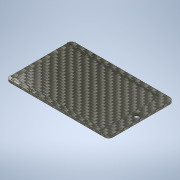
# Autodesk Inventor part: magnet card bottom
Saved by Autodesk Inventor 2020 (Build 240168000, 168)
## iProperties
Created: 2019-06-07
Part Number: magnet card bottom
Material: Generic
Document SubType Name: Modeling
Designer: kangh
Density: 1 g/cm^3
Appearance: Carbon Fiber 1
Author: kangh
Autodesk Inventor part; units mm, degrees
ref_plane "YZ Plane" through (0, 0, 0) normal (1, 0, 0) x (0, 1, 0)
ref_plane "XZ Plane" through (0, 0, 0) normal (0, 1, 0) x (-1, 0, 0)
ref_plane "XY Plane" through (0, 0, 0) normal (0, 0, 1) x (1, 0, 0)
sketch "Sketch1" plane through (0, 0, 0) normal (0, 1, 0) x (-1, 0, 0)
  line L0 (0, 0) -> (85.6, 0)
  line L1 (85.6, 0) -> (85.6, 53.98)
  line L2 (85.6, 53.98) -> (0, 53.98)
  line L3 (0, 53.98) -> (0, 0)
  line L4 (0, 53.98) -> (0, 50.8)
  line L5 (0, 50.8) -> (3.18, 50.8)
  circle A0 centre (3.18, 50.8) radius 3.18
  line L6 (85.6, 53.98) -> (85.6, 57.98)
  line L7 (85.6, 57.98) -> (0, 57.98)
  line L8 (0, 57.98) -> (-9, 57.98)
  line L9 (-9, 57.98) -> (-9, 0)
  line L10 (-9, 0) -> (0, 0)
  line L11 (0, 26.99) -> (-4.5, 26.99)
  circle A1 centre (-4.5, 26.99) radius 2.5
  line L12 (85.6, 55.98) -> (65.6, 55.98)
  circle A2 centre (65.6, 55.98) radius 1
  line L13 (0, 26.99) -> (85.6, 26.99)
  line L14 (85.6, -4) -> (0, -4)
  line L15 (0, -4) -> (-9, -4)
  circle A3 centre (65.6, -2) radius 1
  line L16 (85.6, -4) -> (85.6, 0)
  line L17 (-9, -4) -> (-9, 0)
  line L18 (85.6, 57.98) -> (88.6, 57.98)
  line L19 (88.6, 57.98) -> (88.6, -4)
  line L20 (88.6, -4) -> (85.6, -4)
  line L21 (85.6, -4) -> (85.6, 57.98)
  line L22 (85.6, 53.98) -> (88.6, 53.98)
  line L23 (85.6, 0) -> (88.6, 0)
  circle A4 centre (3.18, 3.18) radius 3.18
  point P0 (3.18, 0)
  point P1 (0, 3.18)
  point P2 (3.18, 53.98)
  dimension "d0" = 85.6
  dimension "d1" = 53.98
  dimension "d2" = 3.18
  dimension "d3" = 3.18
  dimension "d4" = 4
  dimension "d5" = 9
  dimension "d6" = 5
  dimension "d7" = 20
  dimension "d8" = 2
  dimension "d9" = 3
  constraints: 48 end point, 9 perpendicular, 6 point on line, 5 parallel, 5 symmetric about line, 4 centre point, 3 coincident, 3 horizontal, 3 midpoint, 1 vertical, 5 other
  measures "d0" distance of L2.end L1.end
  measures "d1" distance of L1.end L0.end
  measures "d2" distance of L2.end L4.end
  measures "d3" distance of L4.end L5.end
  measures "d4" distance of L1.end L6.end
  measures "d5" distance of L7.end L8.end
  measures "d6" diameter of A1
  measures "d7" distance of L12.start L12.end
  measures "d8" diameter of A2
  measures "d9" distance of L19.end L20.end
extrude "Extrusion1" add sketch "Sketch1" along normal blind 2 contours L3 A4 L0 | L10 L9 L8 L7 L6 L2 L3 | L0 L16 L14 L15 L17 L10 | L3 L2 A0 | L6 L18 L19 L22
extrude "Extrusion2" add sketch "Sketch1" along normal blind 1 contours A4 L3 L13 L1 L0 | A4 | L3 A0 L2 L1 L13 | A0
extrude "Extrusion3" add sketch "Sketch1" along normal blind 2 contours L23 L19 L20 L16
extrude "Extrusion4" add sketch "Sketch1" along normal blind 1.5 contours L1 L22 L19 L23
fillet "Fillet1" radius 24.13 1 edges at (-85.6, 1.5, 26.99)
fillet "Fillet2" radius 4 4 edges at (-88.6, 1, 57.98) (-88.6, 1, -4) (9, 1, -4) (9, 1, 57.98)
body "Solid1"
